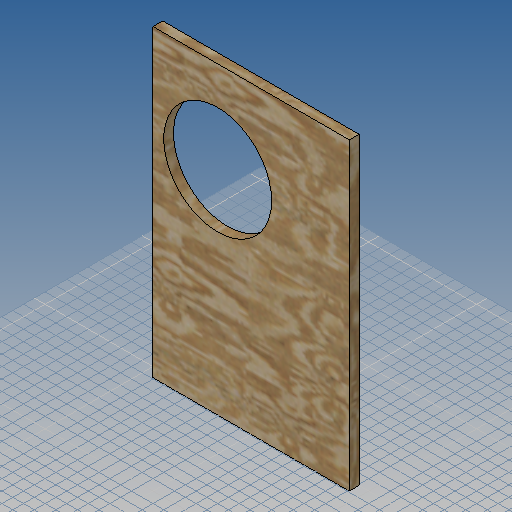
# Autodesk Inventor part: Korpus_Basis
Saved by Autodesk Inventor 2019 (Build 230136000, 136)
## iProperties
Created: 2020-08-02
Part Number: Korpus_Basis
Material: Generisch
Document SubType Name: Modeling
Designer: Stefan
Mass: 3129.84 g
Surface Area: 3924.78 cm^2
Volume: 3129.84 cm^3
Density: 1 g/cm^3
Appearance: Sperrholz - verwittert
Author: Stefan
Autodesk Inventor part; units mm, degrees
ref_plane "YZ Plane" through (0, 0, 0) normal (1, 0, 0) x (0, 1, 0)
ref_plane "XZ Plane" through (0, 0, 0) normal (0, 1, 0) x (-1, 0, 0)
ref_plane "XY Plane" through (0, 0, 0) normal (0, 0, 1) x (1, 0, 0)
sketch "Skizze1" plane through (0, 0, 0) normal (0, 0, 1) x (1, 0, 0)
  line L0 (-182, -282) -> (182, -282)
  line L1 (182, -282) -> (182, 282)
  line L2 (182, 282) -> (-182, 282)
  line L3 (-182, 282) -> (-182, -282)
  line L4 (-182, -282) -> (182, 282) construction
  line L5 (182, -282) -> (-182, 282) construction
  circle A0 centre (-62, 112) radius 100
  point P0 (0, 0)
  point P1 (0, 0)
  dimension "d0" = 364
  dimension "d1" = 564
  dimension "d4" = 200
  dimension "d5" = 170
  dimension "d6" = 120
  constraints: 12 end point, 3 midpoint, 2 parallel, 1 centre point, 1 horizontal, 1 perpendicular
  measures "d0" distance of L1.end L2.end
  measures "d1" distance of L2.end L0.start
  measures "d4" diameter of A0
  measures "d5" distance from line of A0.centre L2
  measures "d6" distance from line of L3 A0.centre
extrude "Extrusion1" add sketch "Skizze1" along normal blind 18
equation "\"d0\" = case_width - 2 * case_thickness"
equation "\"d1\" = case_depth - 2 * case_thickness"
equation "\"d4\" = kg_diameter"
equation "\"d2\" = case_thickness"
equation "\"kg_diameter\" = 200"
equation "\"kg_thickness\" = 4.9"
equation "\"ht_thickness\" = 1.9"
equation "\"case_thickness\" = 18"
equation "\"inner_thickness\" = 15"
equation "\"gap_fit\" = 0.1"
equation "\"gap_slide\" = 0.2"
equation "\"gap_air\" = 1"
equation "\"bore_diameter\" = 73"
equation "\"mdf_thickness\" = 6"
equation "\"tape_width\" = 15"
equation "\"tape_thickness\" = 3"
equation "\"inner_depth\" = 255"
equation "\"case_width\" = 400"
equation "\"case_depth\" = 600"
